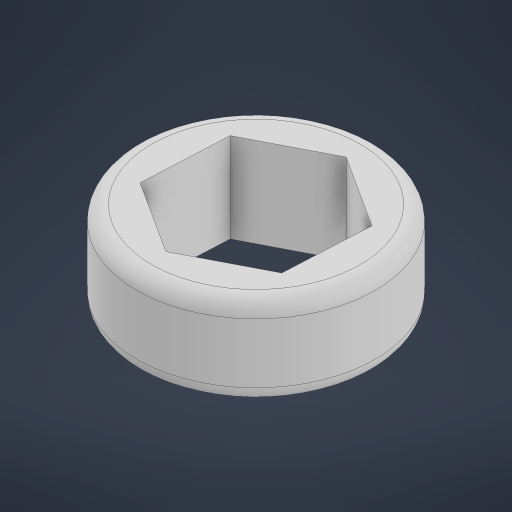
# Autodesk Inventor part: oc5mm
Saved by Autodesk Inventor 2023 (Build 270158000, 158)
## iProperties
Created: 2023-09-13
Part Number: oc5mm
Material: Generic
Document SubType Name: Modeling
Designer: philo
Density: 1 g/cm^3
Appearance: Default
Author: philo
Autodesk Inventor part; units mm, degrees
ref_plane "YZ Plane" through (0, 0, 0) normal (1, 0, 0) x (0, 1, 0)
ref_plane "XZ Plane" through (0, 0, 0) normal (0, 1, 0) x (-1, 0, 0)
ref_plane "XY Plane" through (0, 0, 0) normal (0, 0, 1) x (1, 0, 0)
sketch "Sketch1" plane through (0, 0, 0) normal (0, 1, 0) x (-1, 0, 0)
  circle A0 centre (0, 0) radius 4
  line L0 (2.4276, -1.5621) -> (-0.1391, -2.8834)
  line L1 (-0.1391, -2.8834) -> (-2.5666, -1.3213)
  line L2 (-2.5666, -1.3213) -> (-2.4276, 1.5621)
  line L3 (-2.4276, 1.5621) -> (0.1391, 2.8834)
  line L4 (0.1391, 2.8834) -> (2.5666, 1.3213)
  line L5 (2.5666, 1.3213) -> (2.4276, -1.5621)
  dimension "d0" = 8
  dimension "d1" = 2.5
  constraints: 12 end point, 2 coincident, 1 centre point, 13 other
  measures "d0" diameter of A0
  measures "d1" distance from line of point (0, 0) L5
extrude "Extrusion1" add sketch "Sketch1" along normal blind 3
fillet "Fillet1" radius 0.5 2 edges at (4, 3, 0) (4, 0, 0)
body "Solid1"
